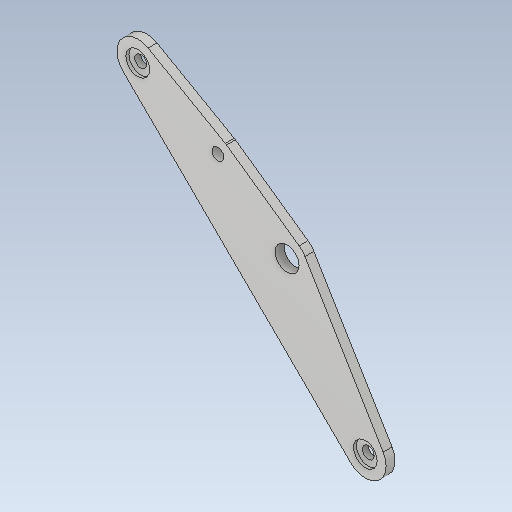
# Autodesk Inventor part: アーム左フレーム
Saved by Autodesk Inventor 2020 (Build 240168000, 168)
## iProperties
Created: 2019-12-03
Part Number: アーム左フレーム
Material: アルミニウム 2014-T4
Document SubType Name: Modeling
Designer: tanjihayato
Density: 2.8 g/cm^3
Appearance: サテン
Mass: 19.323 g
Surface Area: 56.5339 cm^2
Volume: 6.90106 cm^3
Author: tanjihayato
Autodesk Inventor part; units mm, degrees
ref_plane "YZ Plane" through (0, 0, 0) normal (1, 0, 0) x (0, 1, 0)
ref_plane "XZ Plane" through (0, 0, 0) normal (0, 1, 0) x (-1, 0, 0)
ref_plane "XY Plane" through (0, 0, 0) normal (0, 0, 1) x (1, 0, 0)
sketch "スケッチ1" plane through (0, 0, 0) normal (0, 0, 1) x (1, 0, 0)
  circle A0 centre (3.7003, 45.5208) radius 4
  circle A1 centre (80.4159, -30.3183) radius 4
  circle A2 centre (80.4159, -30.3183) radius 2
  circle A3 centre (3.7003, 45.5208) radius 2
  circle A4 centre (30.7326, 32.4678) radius 2
  circle A5 centre (54.047, 13.5882) radius 4.025
  arc A6 (7.1573, 51.6076) -> (-1.2209, 40.5427) centre (3.7003, 45.5208) ccw
  arc A7 (75.4946, -35.2964) -> (86.4186, -26.7173) centre (80.4159, -30.3183) ccw
  arc A8 (60.0712, 17.2021) -> (58.0894, 19.3336) centre (54.047, 13.5882) ccw
  arc A9 (33.6098, 36.5571) -> (33.2019, 36.8155) centre (30.7326, 32.4678) ccw
  line L0 (7.1573, 51.6076) -> (33.2019, 36.8155)
  line L1 (33.6098, 36.5571) -> (58.0894, 19.3336)
  line L2 (60.0712, 17.2021) -> (86.4186, -26.7173)
  line L3 (-1.2209, 40.5427) -> (75.4946, -35.2964)
  point P0 (0, 0)
  point P1 (0, 0)
  dimension "d0" = 3
  dimension "d1" = 3
  dimension "d2" = 3
  dimension "d3" = 3
  constraints: 10 centre point, 8 end point, 8 point on circle, 8 tangent
  measures "d0" radial gap between concentric circles of A0 A6
  measures "d1" radial gap between concentric circles of A1 A7
  measures "d2" radial gap between concentric circles of A5 A8
  measures "d3" radial gap between concentric circles of A4 A9
extrude "押し出し1" add sketch "スケッチ1" along normal blind 3 contours L0 A9 L1 A8 L2 A7 L3 A6
extrude "押し出し2" add sketch "スケッチ1" along normal blind 2 contours A0 | A1
